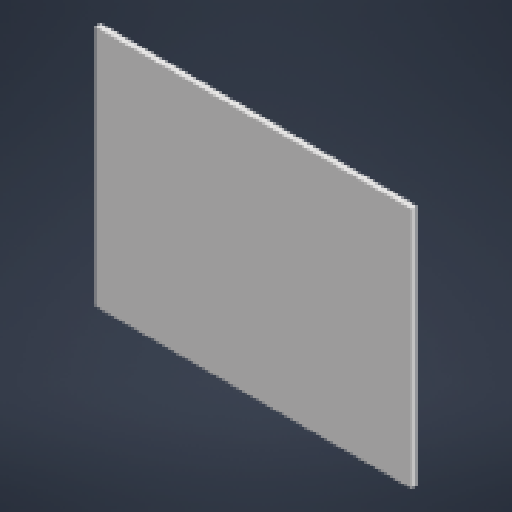
# Autodesk Inventor part: Pieza3
Saved by Autodesk Inventor 2026.1 (Build 301233020, 233B)
## iProperties
Created: 2026-05-06
Part Number: Pieza3
Material: Genérico
Document SubType Name: Modeling
Designer: OlmesTech
Density: 1 g/cm^3
Appearance: Valor por defecto
Author: OlmesTech
Autodesk Inventor part; units mm, degrees
ref_plane "YZ Plane" through (0, 0, 0) normal (1, 0, 0) x (0, 1, 0)
ref_plane "XZ Plane" through (0, 0, 0) normal (0, 1, 0) x (-1, 0, 0)
ref_plane "XY Plane" through (0, 0, 0) normal (0, 0, 1) x (1, 0, 0)
sketch "Boceto1" plane through (0, 0, 0) normal (0, 0, 1) x (1, 0, 0)
  line L0 (0, 3) -> (167, 3) projected
  line L1 (0, -127) -> (0, 0) projected
  line L2 (0, 0) -> (0, 3) projected
  line L3 (170, -127) -> (3, -127) projected
  line L4 (3, -127) -> (0, -127) projected
  line L5 (170, -124) -> (170, -127) projected
  line L6 (170, 3) -> (170, -124) projected
  line L7 (167, 3) -> (170, 3) projected
extrude "Extrusión1" add sketch "Boceto1" along normal blind 3
